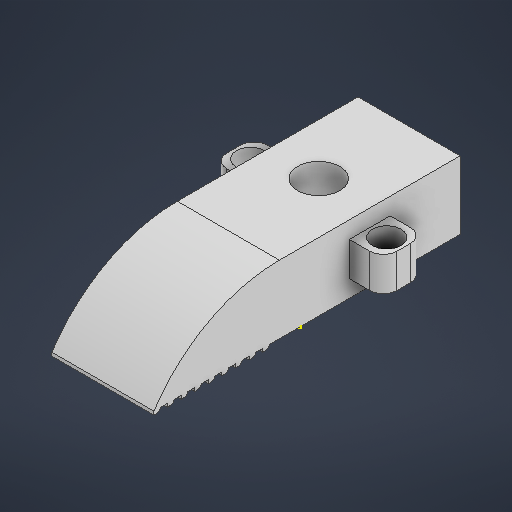
# Autodesk Inventor part: garrasolta
Saved by Autodesk Inventor 2026.1 (Build 301233020, 233B)
## iProperties
Created: 2025-11-06
Part Number: garrasolta
Material: Genérico
Document SubType Name: Modeling
Designer: luska
Density: 1 g/cm^3
Appearance: Padrão
Author: luska
Autodesk Inventor part; units mm, degrees
ref_plane "YZ Plane" through (0, 0, 0) normal (1, 0, 0) x (0, 1, 0)
ref_plane "XZ Plane" through (0, 0, 0) normal (0, 1, 0) x (-1, 0, 0)
ref_plane "XY Plane" through (0, 0, 0) normal (0, 0, 1) x (1, 0, 0)
sketch "Esboço1" plane through (0, 0, 0) normal (0, 1, 0) x (-1, 0, 0)
  line L0 (-4.1047, 21.5372) -> (-19.1047, 21.5372)
  line L1 (-19.1047, 21.5372) -> (-19.1047, -23.4628)
  line L2 (-19.1047, -23.4628) -> (-4.1047, -23.4628)
  line L3 (-4.1047, -23.4628) -> (-4.1047, 21.5372)
  point P0 (0, 0)
  constraints: 8 end point, 2 parallel, 1 horizontal, 1 perpendicular
extrude "Extrusão1" add sketch "Esboço1" along normal blind 10
fillet "Arredondamento1" radius 22 1 edges at (11.6047, 10, 21.5372)
sketch "Esboço2" plane through (0, 10, 0) normal (0, 1, 0) x (1, 0, 0)
  circle A0 centre (11.6047, 10.1828) radius 3.1
  line L0 (19.1047, 23.4628) -> (4.1047, 23.4628) projected
  line L1 (19.1047, -3.0981) -> (4.1047, -3.0981) projected
  line L2 (19.1047, -3.0981) -> (19.1047, 23.4628) projected
  line L3 (4.1047, 23.4628) -> (4.1047, -3.0981) projected
  line L4 (4.1047, -21.5372) -> (19.1047, -21.5372) projected
  point P0 (0, 0)
  point P1 (4.1047, 10.1824)
  dimension "d5" = 6.2
  dimension "d6" = 26.5609
  dimension "d7" = 13.28
  dimension "d8" = 15
  dimension "d9" = 7.5
  dimension "d10" = 18.4391
  constraints: 1 centre point, 1 midpoint
  measures "d5" diameter of A0
  measures "d6" distance between parallel lines of L0 L1
  measures "d7" distance from line of A0.centre L0
  measures "d8" distance between parallel lines of L2 L3
  measures "d9" distance of point (4.105, 10.182) A0.centre
  measures "d10" distance between parallel lines of L4 L1
extrude "Extrusão2" cut sketch "Esboço2" against normal blind 10 contours A0
sketch "Esboço3" plane through (4.1047, 0, -23.4628) normal (-1, 0, 0) x (0, 0, 1)
  line L0 (10.28, 7.5) -> (16.28, 7.5)
  line L1 (16.28, 7.5) -> (16.28, 2.5)
  line L2 (16.28, 2.5) -> (10.28, 2.5)
  line L3 (10.28, 2.5) -> (10.28, 7.5)
  line L4 (0, 0) -> (0, 10) projected
  line L5 (0, 10) -> (26.5609, 10) projected
  point P0 (23.4628, 0)
  point P1 (0, 5)
  point P2 (10.28, 5)
  point P3 (16.28, 5)
  point P4 (13.28, 7.5)
  dimension "d13" = 10.28
  dimension "d14" = 6
  dimension "d15" = 5
  dimension "d16" = 2.5
  constraints: 8 end point, 4 midpoint, 2 parallel, 1 horizontal, 1 perpendicular
  measures "d13" distance of point (0, 5) point (10.28, 5)
  measures "d14" distance from line of L3 point (16.28, 5)
  measures "d15" distance from line of L2 point (13.28, 7.5)
  measures "d16" distance between parallel lines of L5 L0
extrude "Extrusão3" add sketch "Esboço3" along normal blind 5
sketch "Esboço4" plane through (19.1047, 0, -23.4628) normal (1, 0, 0) x (0, 0, -1)
  point P0 (-23.4628, 0)
sketch "Esboço5" plane through (19.1047, 0, -23.4628) normal (1, 0, 0) x (0, 0, -1)
  line L0 (-10.28, 7.5) -> (-16.28, 7.5)
  line L1 (-16.28, 7.5) -> (-16.28, 2.5)
  line L2 (-16.28, 2.5) -> (-10.28, 2.5)
  line L3 (-10.28, 2.5) -> (-10.28, 7.5)
  line L4 (0, 0) -> (0, 10) projected
  line L5 (-26.5609, 10) -> (0, 10) projected
  point P0 (-23.4628, 0)
  point P1 (0, 5)
  point P2 (-10.28, 5)
  point P3 (-13.28, 2.5)
  dimension "d19" = 10.28
  dimension "d20" = 6
  dimension "d21" = 5
  dimension "d22" = 2.5
  constraints: 8 end point, 3 midpoint, 2 parallel, 1 horizontal, 1 perpendicular
  measures "d19" distance of point (0, 5) point (-10.28, 5)
  measures "d20" distance between parallel lines of L1 L3
  measures "d21" distance from line of point (-13.28, 2.5) L0
  measures "d22" distance between parallel lines of L5 L0
extrude "Extrusão4" add sketch "Esboço5" along normal blind 5
sketch "Esboço6" plane through (4.1047, 7.5, -7.1828) normal (0, 1, 0) x (1, 0, 0)
  circle A0 centre (-2.5, 3) radius 2.1
  circle A1 centre (17.5, 3) radius 2.1
  line L0 (0, 6) -> (0, 0) projected
  line L1 (0, 6) -> (-5, 6) projected
  line L2 (15, 0) -> (15, 6) projected
  line L3 (15, 6) -> (20, 6) projected
  point P0 (-4.1047, -7.1828)
  point P1 (15, 3)
  dimension "d25" = 4.2
  dimension "d26" = 4.2
  dimension "d27" = 2.5
  dimension "d28" = 3
  dimension "d29" = 2.5
  dimension "d30" = 3
  constraints: 2 centre point, 1 midpoint
  measures "d25" diameter of A0
  measures "d26" diameter of A1
  measures "d27" distance from line of L0 A0.centre
  measures "d28" distance from line of A0.centre L1
  measures "d29" distance of point (15, 3) A1.centre
  measures "d30" distance from line of L3 A1.centre
extrude "Extrusão5" cut sketch "Esboço6" against normal blind 5
fillet "Arredondamento2" radius 2 4 edges at (24.1047, 5, -13.1828) (24.1047, 5, -7.1828) (-0.8953, 5, -13.1828) (-0.8953, 5, -7.1828)
sketch "Esboço7" plane through (0, 0, 0) normal (0, -1, 0) x (1, 0, 0)
  line L0 (4.1047, 21.5372) -> (19.1047, 21.5372) projected
  line L1 (4.1047, -23.4628) -> (4.1047, 21.5372) projected
  line L2 (19.1047, 21.5372) -> (4.1047, 21.5372)
  line L3 (4.1047, 21.5372) -> (4.1047, 20.5372)
  line L4 (4.1047, 20.5372) -> (19.1047, 20.5372)
  line L5 (19.1047, 20.5372) -> (19.1047, 21.5372)
  line L6 (11.6047, 3.1072) -> (11.6047, 20.5372)
  line L7 (19.1047, 20.5372) -> (4.1047, 20.5372)
  line L8 (4.1047, 20.5372) -> (4.1047, 19.5372)
  line L9 (4.1047, 19.5372) -> (19.1047, 19.5372)
  line L10 (19.1047, 19.5372) -> (19.1047, 20.5372)
  line L11 (19.1047, 19.5372) -> (4.1047, 19.5372)
  line L12 (4.1047, 19.5372) -> (4.1047, 18.5372)
  line L13 (4.1047, 18.5372) -> (19.1047, 18.5372)
  line L14 (19.1047, 18.5372) -> (19.1047, 19.5372)
  line L15 (19.1047, 18.5372) -> (4.1047, 18.5372)
  line L16 (4.1047, 18.5372) -> (4.1047, 17.5372)
  line L17 (4.1047, 17.5372) -> (19.1047, 17.5372)
  line L18 (19.1047, 17.5372) -> (19.1047, 18.5372)
  line L19 (19.1047, 17.5372) -> (4.1047, 17.5372)
  line L20 (4.1047, 17.5372) -> (4.1047, 16.5372)
  line L21 (4.1047, 16.5372) -> (19.1047, 16.5372)
  line L22 (19.1047, 16.5372) -> (19.1047, 17.5372)
  line L23 (19.1047, 16.5372) -> (4.1047, 16.5372)
  line L24 (4.1047, 16.5372) -> (4.1047, 15.5372)
  line L25 (4.1047, 15.5372) -> (19.1047, 15.5372)
  line L26 (19.1047, 15.5372) -> (19.1047, 16.5372)
  line L27 (19.1047, 15.5372) -> (4.1047, 15.5372)
  line L28 (4.1047, 15.5372) -> (4.1047, 14.5372)
  line L29 (4.1047, 14.5372) -> (19.1047, 14.5372)
  line L30 (19.1047, 14.5372) -> (19.1047, 15.5372)
  line L31 (19.1047, 14.5372) -> (4.1047, 14.5372)
  line L32 (4.1047, 14.5372) -> (4.1047, 13.5372)
  line L33 (4.1047, 13.5372) -> (19.1047, 13.5372)
  line L34 (19.1047, 13.5372) -> (19.1047, 14.5372)
  line L35 (19.1047, 13.5372) -> (4.1047, 13.5372)
  line L36 (4.1047, 13.5372) -> (4.1047, 12.5372)
  line L37 (4.1047, 12.5372) -> (19.1047, 12.5372)
  line L38 (19.1047, 12.5372) -> (19.1047, 13.5372)
  line L39 (19.1047, 12.5372) -> (4.1047, 12.5372)
  line L40 (4.1047, 12.5372) -> (4.1047, 11.5372)
  line L41 (4.1047, 11.5372) -> (19.1047, 11.5372)
  line L42 (19.1047, 11.5372) -> (19.1047, 12.5372)
  line L43 (19.1047, 11.5372) -> (4.1047, 11.5372)
  line L44 (4.1047, 11.5372) -> (4.1047, 10.5372)
  line L45 (4.1047, 10.5372) -> (19.1047, 10.5372)
  line L46 (19.1047, 10.5372) -> (19.1047, 11.5372)
  line L47 (19.1047, 10.5372) -> (4.1047, 10.5372)
  line L48 (4.1047, 10.5372) -> (4.1047, 9.5372)
  line L49 (4.1047, 9.5372) -> (19.1047, 9.5372)
  line L50 (19.1047, 9.5372) -> (19.1047, 10.5372)
  line L51 (19.1047, 9.5372) -> (4.1047, 9.5372)
  line L52 (4.1047, 9.5372) -> (4.1047, 8.5372)
  line L53 (4.1047, 8.5372) -> (19.1047, 8.5372)
  line L54 (19.1047, 8.5372) -> (19.1047, 9.5372)
  line L55 (19.1047, 8.5372) -> (4.1047, 8.5372)
  line L56 (4.1047, 8.5372) -> (4.1047, 7.5372)
  line L57 (4.1047, 7.5372) -> (19.1047, 7.5372)
  line L58 (19.1047, 7.5372) -> (19.1047, 8.5372)
  line L59 (19.1047, 7.5372) -> (4.1047, 7.5372)
  line L60 (4.1047, 7.5372) -> (4.1047, 6.5372)
  line L61 (4.1047, 6.5372) -> (19.1047, 6.5372)
  line L62 (19.1047, 6.5372) -> (19.1047, 7.5372)
  line L63 (19.1047, 6.5372) -> (4.1047, 6.5372)
  line L64 (4.1047, 6.5372) -> (4.1047, 5.5372)
  line L65 (4.1047, 5.5372) -> (19.1047, 5.5372)
  line L66 (19.1047, 5.5372) -> (19.1047, 6.5372)
  line L67 (19.1047, 5.5372) -> (4.1047, 5.5372)
  line L68 (4.1047, 5.5372) -> (4.1047, 4.5372)
  line L69 (4.1047, 4.5372) -> (19.1047, 4.5372)
  line L70 (19.1047, 4.5372) -> (19.1047, 5.5372)
  point P0 (0, 0)
  point P1 (11.6047, 19.5372)
  point P2 (11.6047, 18.5372)
  point P3 (11.6047, 17.5372)
  point P4 (11.6047, 16.5372)
  point P5 (11.6047, 15.5372)
  point P6 (11.6047, 14.5372)
  point P7 (11.6047, 13.5372)
  point P8 (11.6047, 12.5372)
  point P9 (11.6047, 11.5372)
  point P10 (11.6047, 10.5372)
  point P11 (11.6047, 9.5372)
  point P12 (11.6047, 8.5372)
  point P13 (11.6047, 7.5372)
  point P14 (11.6047, 6.5372)
  point P15 (11.6047, 5.5372)
  point P16 (11.6047, 4.5372)
  dimension "d34" = 1
  dimension "d35" = 17.43
  dimension "d39" = 1
  constraints: 138 end point, 2 parallel, 1 horizontal, 1 midpoint, 1 perpendicular, 1 point on line, 1 vertical, 144 other
  measures "d34" distance between parallel lines of L0 L4
  measures "d35" distance of L6.end L6.start
  measures "d39" distance of L3.end L8.end
extrude "Extrusão6" add sketch "Esboço7" along normal blind 0.5 contours L0 L5 L4 L1 | L9 L6 L13 L1 | L14 L13 L6 L9 | L17 L6 L21 L1 | L22 L21 L6 L17 | L25 L6 L29 L1 | L30 L29 L6 L25 | L33 L6 L37 L1 | L38 L37 L6 L33 | L41 L6 L45 L1 | L46 L45 L6 L41 | L49 L6 L53 L1 | L54 L53 L6 L49 | L57 L6 L61 L1 | L62 L61 L6 L57 | L65 L6 L69 L1 | L70 L69 L6 L65
fillet "Arredondamento3" radius 0.7 9 edges at (11.6047, -0.5, 4.5372) (11.6047, -0.5, 6.5372) (11.6047, -0.5, 8.5372) (11.6047, -0.5, 10.5372) (11.6047, -0.5, 12.5372) (11.6047, -0.5, 14.5372) (11.6047, -0.5, 16.5372) (11.6047, -0.5, 18.5372) (11.6047, -0.5, 20.5372)
sketch "Esboço8" plane through (0, 0, 0) normal (0, -1, 0) x (1, 0, 0)
  point P0 (0, 0)
sketch "Esboço9" plane through (0, 0, 0) normal (0, -1, 0) x (1, 0, 0)
  line L0 (9.144, -14.4589) -> (6.6591, -10.2107)
  line L1 (6.6591, -10.2107) -> (9.0958, -5.9346)
  line L2 (9.0958, -5.9346) -> (14.0172, -5.9068)
  line L3 (14.0172, -5.9068) -> (16.5021, -10.155)
  line L4 (16.5021, -10.155) -> (14.0655, -14.431)
  line L5 (14.0655, -14.431) -> (9.144, -14.4589)
  line L6 (19.1047, -23.4628) -> (4.1047, -23.4628) projected
  point P0 (0, 0)
  point P1 (11.5806, -10.1828)
  dimension "d47" = 0.324
  dimension "d48" = 13.28
  constraints: 12 end point, 13 other
  measures "d47" angle of L6 L5
  measures "d48" distance from line of L6 point (11.581, -10.183)
extrude "Extrusão7" cut sketch "Esboço9" against normal blind 5
